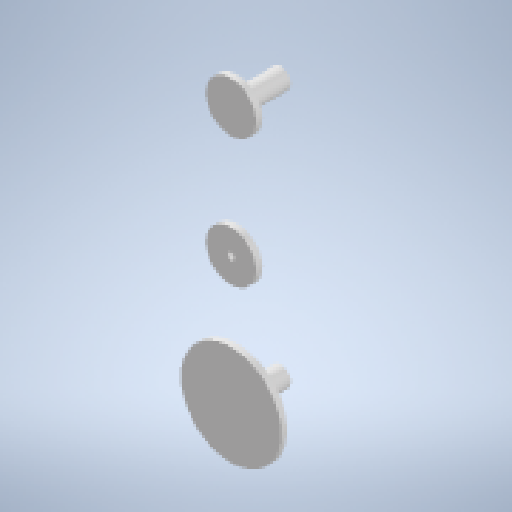
# Autodesk Inventor part: gears
Saved by Autodesk Inventor 2023 (Build 270158000, 158)
## iProperties
Created: 2022-09-15
Part Number: gears
Material: Generic
Document SubType Name: Modeling
Designer: simon
Density: 1 g/cm^3
Appearance: Default
Author: simon
Autodesk Inventor part; units mm, degrees
ref_plane "YZ Plane" through (0, 0, 0) normal (1, 0, 0) x (0, 1, 0)
ref_plane "XZ Plane" through (0, 0, 0) normal (0, 1, 0) x (-1, 0, 0)
ref_plane "XY Plane" through (0, 0, 0) normal (0, 0, 1) x (1, 0, 0)
sketch "Sketch1" plane through (0, 0, 0) normal (0, 0, 1) x (1, 0, 0)
  circle A0 centre (0, 0) radius 2.5 projected
  circle A1 centre (0, 0) radius 2.5 projected
  circle A2 centre (0, 0) radius 12.5 projected
  circle A3 centre (0, 0) radius 2.75
  circle A4 centre (0, 0) radius 12.5
  circle A5 centre (0, -103) radius 8 projected
  circle A6 centre (0, -103) radius 8
  circle A7 centre (0, -103) radius 40
  circle A8 centre (0, 0) radius 20
  circle A9 centre (0, 103) radius 8 projected
  circle A10 centre (0, 103) radius 20
  dimension "d0" = 5.5
  dimension "d1" = 80
  dimension "d2" = 25
  dimension "d3" = 40
  dimension "d4" = 40
  constraints: 6 centre point, 6 coincident, 2 concentric
  measures "d0" diameter of A3
  measures "d1" diameter of A7
  measures "d2" diameter of A2
  measures "d3" diameter of A10
  measures "d4" diameter of A8
extrude "Extrusion1" add sketch "Sketch1" along normal blind 5 contours A2 | A5 | A7 | A8 | A9 | A10
extrude "Extrusion2" add sketch "Sketch1" against normal blind 35 contours A5 | A9
body "Solid1"
